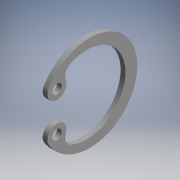
# Autodesk Inventor part: LH-RRING-C-INT-S-19
Saved by Autodesk Inventor 2017.3 (Build 213256000, 256)
## iProperties
Part Number: LH-RRING-C-INT-S-19
Material: Generic
Catalog Web Link: www.cadenas.de
Description: LH_RRING_C_INT-Retaining Rings - C  (Internal)
Vendor: MISUMI
Document SubType Name: Modeling
Designer: partserver
Manufacturer: MISUMI
Mass: 0.110311 g
Surface Area: 3.39751 cm^2
Volume: 0.110311 cm^3
Density: 1 g/cm^3
Appearance: PSOLRGB-192-192-192
Category: PARTsolutions
Company: MISUMI
Title: LH-RRING-C-INT-S-19
Author: Cadenas PARTsolutions
Comments: Retaining Rings - C  (Internal)
PSOL_IDENT_0: {$CADENAS_DATA\23d-libs\misumi\metric\04_linear_bushings\04_accessories\lh_rring_c_int.prj},189 {VTY
PSOL_IDENT_1: P=3D},{NB=LH-RRING-C-INT-S-19},{LINA=LH-RRING-C-INT-S-19},{NN=LH_RRING_C_INT},{DATE=30.03.2018 01:15
PSOL_IDENT_2: :19},{GEOMDATE=18.03.2015 00:00:00},{VERSION=},{LINEID=380},{WBVAR=TS},{WBNUMERIC=}  {NB=LH-RRING-C-
PSOL_IDENT_3: INT-S-19},{LINA=LH-RRING-C-INT-S-19},{KT=DUMMY},{PN=LH-RRING-C-INT-S-19},{TYPE=LH-RRING-C-INT-S},{TS=
PSOL_IDENT_4: S},{NO=19},{TT=1.00},{BB=2.5},{AA=4.0},{DD0=2.0},{DD2=20.0},{A=8.3}
NB: LH-RRING-C-INT-S-19
NN: LH_RRING_C_INT
NT: Retaining Rings - C  (Internal)
NBSYN: $PN.
LINA: LH-RRING-C-INT-S-19
CATALOG: Misumi
PN: LH-RRING-C-INT-S-19
TS: Standard Type
NO: 19
TT: 1
BB: 2.5
AA: 4
DD0: 2
DD2: 20
A: 8.3
SUPPLIER: MISUMI
ARTICLENO: LH-RRING-C-INT-S-19
BOMINFO: LH-RRING-C-INT-S-19
CREATOR: CADENAS GmbH
Autodesk Inventor part; units mm, degrees
ref_plane "YZ Plane" through (0, 0, 0) normal (1, 0, 0) x (0, 1, 0)
ref_plane "XZ Plane" through (0, 0, 0) normal (0, 1, 0) x (-1, 0, 0)
ref_plane "XY Plane" through (0, 0, 0) normal (0, 0, 1) x (1, 0, 0)
sketch "Sketch_3" plane through (0, 0, 0) normal (1, 0, 0) x (0, 1, 0)
  arc A0 (-8.5493, -5.1875) -> (-8.5493, 5.1875) centre (0, 0) ccw
  arc A1 (-8.5493, 5.1875) -> (-7.4165, 2.2351) centre (-6.8394, 4.15) ccw
  arc A2 (-7.4165, 2.2351) -> (-4.975, 4.874) centre (-6.8394, 4.15) ccw
  arc A3 (-3.9223, 7.4259) -> (-4.975, 4.874) centre (-3.1107, 5.5979) ccw
  arc A4 (-3.9223, -7.4259) -> (-3.9223, 7.4259) centre (-0.625, 0) ccw
  arc A5 (-4.975, -4.874) -> (-3.9223, -7.4259) centre (-3.1107, -5.5979) ccw
  arc A6 (-4.975, -4.874) -> (-7.4165, -2.2351) centre (-6.8394, -4.15) ccw
  arc A7 (-7.4165, -2.2351) -> (-8.5493, -5.1875) centre (-6.8394, -4.15) ccw
  circle A8 centre (-6.8394, -4.15) radius 1
  circle A9 centre (-6.8394, 4.15) radius 1
  constraints: 16 point on circle, 10 centre point
extrude "Extrusion1" add sketch "Sketch_3" along normal mid plane 1
ref_plane "rr_XY" through (-0.5, 0, 0) normal (1, 0, 0) x (0, 0, -1)
ref_plane "rr_YZ" through (-0.5, 0, 0) normal (0, 0, -1) x (0, 1, 0)
ref_plane "rr_ZX" through (-0.5, 0, 0) normal (0, 1, 0) x (1, 0, 0)
body "Solid1"
